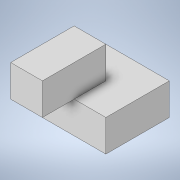
# Autodesk Inventor part: Square with Lobe
Saved by Autodesk Inventor 2020 (Build 240168000, 168)
## iProperties
Created: 2019-12-20
Part Number: Square with Lobe
Material: Generic
Document SubType Name: Modeling
Designer: Corey
Density: 1 g/cm^3
Appearance: Default
Author: Corey
Autodesk Inventor part; units mm, degrees
ref_plane "YZ Plane" through (0, 0, 0) normal (1, 0, 0) x (0, 1, 0)
ref_plane "XZ Plane" through (0, 0, 0) normal (0, 1, 0) x (-1, 0, 0)
ref_plane "XY Plane" through (0, 0, 0) normal (0, 0, 1) x (1, 0, 0)
sketch "Sketch1" plane through (0, 0, 0) normal (0, 1, 0) x (-1, 0, 0)
  line L0 (0, 0) -> (38.1, 0)
  line L1 (38.1, 0) -> (38.1, -38.1)
  line L2 (38.1, -38.1) -> (0, -38.1)
  line L3 (0, -38.1) -> (0, 0)
  line L4 (38.1, -38.1) -> (19.05, -38.1)
  line L5 (38.1, -19.05) -> (38.1, -38.1)
  line L6 (38.1, -38.1) -> (19.05, -38.1)
  line L7 (19.05, -19.05) -> (38.1, -19.05)
  line L8 (38.1, -19.05) -> (38.1, 19.05)
  line L9 (38.1, 19.05) -> (19.05, 19.05)
  line L10 (19.05, 19.05) -> (19.05, -19.05)
  point P0 (19.05, 0)
  dimension "d0" = 38.1
  dimension "d1" = 38.1
  dimension "d14" = 19.05
  dimension "d15" = 38.1
  constraints: 22 end point, 4 horizontal, 4 parallel, 2 perpendicular
  measures "d0" distance of L1.end L2.end
  measures "d1" distance of L0.end L1.end
  measures "d14" distance of L9.end L8.end
  measures "d15" distance of L8.end L7.end
extrude "Extrusion5" add sketch "Sketch1" along normal blind 19.05 contours L0 L10 L7 L1 L2 L3
extrude "Extrusion6" add sketch "Sketch1" along normal blind 38.1 contours L0 L1 L7 L10
extrude "Extrusion7" add sketch "Sketch1" along normal blind 38.1 contours L10 L9 L8 L0
extrude "Extrusion8" cut sketch "Sketch1" along normal blind 19.05 contours L10 L9 L8 L0
body "Solid2"
